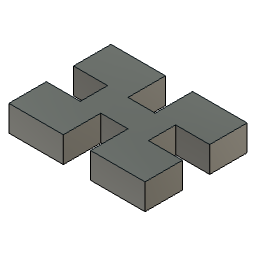
connector (Autodesk Fusion 360 design; units mm, degrees)
Autodesk Fusion 360 part; units mm, degrees
sketch "Sketch1" plane through (0, 0, 0) normal (0, 0, 1) x (1, 0, 0)
  line L0 (0, 0) -> (20, 0)
  line L1 (20, 0) -> (20, 15)
  line L2 (20, 15) -> (0, 15)
  line L3 (0, 15) -> (0, 0)
  line L4 (15, 0) -> (15, 15)
  line L5 (5, 0) -> (5, 15)
  line L6 (0, 7.5) -> (20, 7.5) construction
  line L7 (0, 5.5) -> (20, 5.5)
  line L8 (0, 9.5) -> (20, 9.5)
  line L9 (10, 15) -> (10, 0) construction
  line L10 (8, 15) -> (8, 0)
  line L11 (12, 15) -> (12, 0)
  dimension "d1" = 2
  dimension "d2" = 2
  constraint horizontal L0
  constraint vertical L1
  constraint horizontal L2
  constraint vertical L3
  constraint coincident L0.start L3.end
  constraint coincident L0 L4.start
  constraint coincident L2 L4.end
  constraint perpendicular L2 L4
  constraint coincident L0 L5.start
  constraint coincident L2 L5.end
  constraint perpendicular L2 L5
  constraint midpoint L3 L6.start
  constraint midpoint L1 L6.end
  constraint symmetric L6 L7.start L8.start
  constraint symmetric L6 L7.end L8.end
  constraint midpoint L2 L9.start
  constraint midpoint L0 L9.end
  constraint symmetric L9 L10.start L11.start
  constraint symmetric L9 L10.end L11.end
extrude "Extrude1" add sketch "Sketch1" along normal blind 3.8 contours L0 L3 L5 L7 | L0 L5 L7 L10 | L5 L7 L8 L10 | L2 L3 L5 L8 | L0 L4 L7 L11 | L7 L8 L10 L11 | L2 L5 L8 L10 | L0 L1 L4 L7 | L4 L7 L8 L11 | L2 L4 L8 L11 | L1 L2 L4 L8
sketch "Sketch2" plane through (0, 0, 3.8) normal (0, 0, 1) x (-1, 0, 0)
  line L0 (-15, -5.5) -> (-15, -9.5)
  line L1 (-15, -9.5) -> (-20, -9.5)
  line L2 (-20, -9.5) -> (-20, -15)
  line L3 (-20, -15) -> (-12, -15)
  line L4 (-12, -15) -> (-12, -9.5)
  line L5 (-12, -9.5) -> (-8, -9.5)
  line L6 (-8, -9.5) -> (-8, -15)
  line L7 (-8, -15) -> (0, -15)
  line L8 (0, -15) -> (0, -9.5)
  line L9 (0, -9.5) -> (-5, -9.5)
  line L10 (-5, -9.5) -> (-5, -5.5)
  line L11 (-5, -5.5) -> (0, -5.5)
  line L12 (0, -5.5) -> (0, 0)
  line L13 (0, 0) -> (-8, 0)
  line L14 (-8, 0) -> (-8, -5.5)
  line L15 (-8, -5.5) -> (-12, -5.5)
  line L16 (-12, -5.5) -> (-12, 0)
  line L17 (-12, 0) -> (-20, 0)
  line L18 (-20, 0) -> (-20, -5.5)
  line L19 (-20, -5.5) -> (-15, -5.5)
